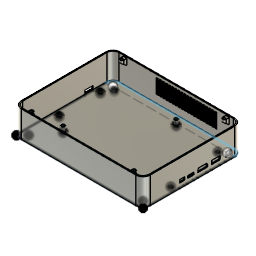
Mini PC Case V7 (Autodesk Fusion 360 design; units mm, degrees)
Autodesk Fusion 360 part; units mm, degrees
note: some values were not read from the file. Set by a fixed rule: which sketch regions a step uses.
sketch "Sketch1" plane through (0, 0, 0) normal (0, 0, 1) x (1, 0, 0)
  line L0 (10, 0) -> (200, 0)
  line L1 (210, 10) -> (210, 150)
  line L2 (210, 150) -> (0, 150) construction
  line L3 (0, 150) -> (0, 10)
  circle A0 centre (119, 146) radius 1.65
  circle A1 centre (191, 143) radius 1.65
  line L4 (-2, 152) -> (-2, 10)
  line L5 (10, -2) -> (200, -2)
  line L6 (212, 10) -> (212, 152)
  circle A2 centre (202, 54) radius 1.65
  circle A3 centre (34.7, 42.5) radius 1.65
  line L7 (210, 143.8) -> (212, 143.8)
  line L8 (210, 135.5) -> (212, 135.5)
  line L9 (210, 126) -> (212, 126)
  line L10 (210, 112) -> (212, 112)
  line L11 (210, 105) -> (212, 105)
  line L12 (210, 89) -> (212, 89)
  line L13 (210, 82.5) -> (212, 82.5)
  line L14 (210, 72) -> (212, 72)
  line L15 (210, 67) -> (212, 67)
  line L16 (210, 59) -> (212, 59)
  circle A4 centre (34.7, 42.5) radius 3
  circle A5 centre (202, 54) radius 3
  circle A6 centre (191, 143) radius 3
  circle A7 centre (119, 146) radius 3
  circle A8 centre (9, 130) radius 1.65
  circle A9 centre (8.6, 62) radius 1.65
  circle A10 centre (9, 130) radius 3
  circle A11 centre (8.6, 62) radius 3
  line L17 (0, 127) -> (-2, 127)
  line L18 (-2, 113.5) -> (0, 113.5)
  circle A12 centre (18, 144.2) radius 4
  line L19 (212, 152) -> (212, 150)
  line L20 (200, 162) -> (10, 162)
  line L21 (-2, 150) -> (-2, 152)
  line L22 (210, 152) -> (210, 150)
  line L23 (200, 160) -> (10, 160)
  line L24 (0, 150) -> (0, 152)
  line L25 (210, 150) -> (210, 152)
  line L26 (0, 150) -> (0, 152)
  arc A13 (200, 0) -> (210, 10) centre (200, 10) ccw
  arc A14 (210, 150) -> (200, 160) centre (200, 150) ccw
  arc A15 (10, 160) -> (0, 150) centre (10, 150) ccw
  arc A16 (0, 10) -> (10, 0) centre (10, 10) ccw
  arc A17 (-2, 10) -> (10, -2) centre (10, 10) ccw
  arc A18 (200, -2) -> (212, 10) centre (200, 10) ccw
  arc A19 (212, 150) -> (200, 162) centre (200, 150) ccw
  arc A20 (10, 162) -> (-2, 150) centre (10, 150) ccw
  point P0 (210, 0)
  dimension "d1" = 210
  dimension "d2" = 150
  dimension "d8" = 3.3
  dimension "d9" = 3.3
  dimension "d24" = 3.3
  dimension "d29" = 3.3
  dimension "d31" = 107.5
  dimension "d33" = 6.2
  dimension "d34" = 14.5
  dimension "d35" = 24
  dimension "d36" = 38
  dimension "d37" = 45
  dimension "d38" = 61
  dimension "d39" = 67.5
  dimension "d40" = 78
  dimension "d41" = 83
  dimension "d42" = 91
  dimension "d46" = 6
  dimension "d48" = 6
  dimension "d49" = 6
  dimension "d50" = 6
  dimension "d53" = 3.3
  dimension "d54" = 20
  dimension "d55" = 9
  dimension "d56" = 3.3
  dimension "d57" = 88
  dimension "d58" = 8.6
  dimension "d59" = 6
  dimension "d60" = 6
  dimension "d65" = 23
  dimension "d66" = 36.5
  dimension "d67" = 8
  dimension "d68" = 18
  dimension "d69" = 5.8
  dimension "d80" = 10
  dimension "d81" = 12
  dimension "d102" = 8
  dimension "d103" = 96
  dimension "d104" = 19
  dimension "d105" = 7
  dimension "d107" = 4
  dimension "d108" = 91
  dimension "d109" = 175.3
  constraint horizontal L0
  constraint vertical L1
  constraint horizontal L2
  constraint vertical L3
  constraint coincident L1 L7.start
  constraint coincident L6 L7.end
  constraint perpendicular L6 L7
  constraint coincident L1 L8.start
  constraint coincident L6 L8.end
  constraint perpendicular L6 L8
  constraint coincident L1 L9.start
  constraint coincident L6 L9.end
  constraint perpendicular L6 L9
  constraint coincident L1 L10.start
  constraint coincident L6 L10.end
  constraint perpendicular L6 L10
  constraint coincident L1 L11.start
  constraint coincident L6 L11.end
  constraint perpendicular L6 L11
  constraint coincident L1 L12.start
  constraint coincident L6 L12.end
  constraint perpendicular L6 L12
  constraint coincident L1 L13.start
  constraint coincident L6 L13.end
  constraint perpendicular L6 L13
  constraint coincident L1 L14.start
  constraint coincident L6 L14.end
  constraint perpendicular L6 L14
  constraint coincident L1 L15.start
  constraint coincident L6 L15.end
  constraint perpendicular L6 L15
  constraint coincident L1 L16.start
  constraint coincident L6 L16.end
  constraint perpendicular L6 L16
  constraint concentric A3 A4
  constraint concentric A2 A5
  constraint concentric A1 A6
  constraint concentric A0 A7
  constraint concentric A8 A10
  constraint concentric A9 A11
  constraint coincident L3 L17.start
  constraint coincident L4 L17.end
  constraint perpendicular L4 L17
  constraint coincident L4 L18.start
  constraint coincident L3 L18.end
  constraint perpendicular L3 L18
  constraint perpendicular L4 L20
  constraint perpendicular L3 L23
  constraint coincident P0 L0
  constraint coincident P0 L1
  constraint tangent L0 A13
  constraint tangent L1 A13
  constraint tangent L22 A14
  constraint tangent L23 A14
  constraint equal A13 A14
  constraint tangent L23 A15
  constraint tangent L24 A15
  constraint equal A13 A15
  constraint coincident origin L0
  constraint coincident origin L3
  constraint tangent L0 A16
  constraint tangent L3 A16
  constraint equal A13 A16
  constraint tangent L4 A17
  constraint tangent L5 A17
  constraint tangent L5 A18
  constraint tangent L6 A18
  constraint equal A17 A18
  constraint tangent L19 A19
  constraint tangent L20 A19
  constraint equal A17 A19
  constraint tangent L20 A20
  constraint tangent L21 A20
  constraint equal A17 A20
  measures "d1" distance of origin P0
  measures "d2" distance of origin L2.end
  measures "d8" diameter of A0
  measures "d9" diameter of A1
  measures "d24" diameter of A2
  measures "d29" diameter of A3
  measures "d31" distance of L2 A3.centre
  measures "d33" distance of L1.end L7
  measures "d34" distance of L1.end L8
  measures "d35" distance of L1.end L9
  measures "d36" distance of L1.end L10
  measures "d37" distance of L1.end L11
  measures "d38" distance of L1.end L12
  measures "d39" distance of L1.end L13
  measures "d40" distance of L1.end L14
  measures "d41" distance of L1.end L15
  measures "d42" distance of L1.end L16
  measures "d46" diameter of A4
  measures "d48" diameter of A5
  measures "d49" diameter of A6
  measures "d50" diameter of A7
  measures "d53" diameter of A8
  measures "d54" distance of L2 A8.centre
  measures "d55" distance of L3 A8.centre
  measures "d56" diameter of A9
  measures "d57" distance of L2 A9.centre
  measures "d58" distance of L3 A9.centre
  measures "d59" diameter of A10
  measures "d60" diameter of A11
  measures "d65" distance of L2 L17
  measures "d66" distance of L2 L18
  measures "d67" diameter of A12
  measures "d68" distance of L3 A12.centre
  measures "d69" distance of L2 A12.centre
  measures "d80" radius of A13
  measures "d81" radius of A17
  measures "d102" distance of L1 A2.centre
  measures "d103" distance of L2 A2.centre
  measures "d104" distance of L1 A1.centre
  measures "d105" distance of L2 A1.centre
  measures "d107" distance of L2 A0.centre
  measures "d108" distance of L1 A0.centre
  measures "d109" distance of L1 A3.centre
extrude "Extrude1" add sketch "Sketch1" along normal blind 2 contours L0 L1 L3 L23 A13 A14 A15 A16 | L0 L1 L3 L4 L5 L6 L16 L18 A13 A16 A17 A18 | L3 L4 L17 L18 | L1 L6 L15 L16 | L1 L3 L4 L6 L7 L17 L20 L23 A14 A15 A19 A20 | L1 L6 L14 L15 | L1 L6 L13 L14 | L1 L6 L12 L13 | L1 L6 L11 L12 | L1 L6 L10 L11 | L1 L6 L7 L8 | L1 L6 L9 L10 | L1 L6 L8 L9 | A0 | A1 | A2 | A3 | A4 | A5 | A6 | A7 | A8 | A9 | A10 | A11
extrude "Extrude2" add sketch "Sketch1" along normal blind 44 contours L0 L1 L3 L4 L5 L6 L16 L18 A13 A16 A17 A18 | L1 L3 L4 L6 L7 L17 L20 L23 A14 A15 A19 A20 | L1 L6 L14 L15 | L1 L6 L12 L13 | L1 L6 L10 L11 | L1 L6 L8 L9
extrude "Extrude3" add sketch "Sketch1" along normal blind 10 contours A4 | A5 | A6 | A7
extrude "Extrude4" add sketch "Sketch1" along normal blind 5 contours A10 | A11
extrude "Extrude8" add sketch "Sketch1" along normal blind 44 and the other way blind -8 contours L3 L4 L17 L18
extrude "Extrude9" add sketch "Sketch1" along normal blind 7 contours L1 L6 L7 L8
extrude "Extrude10" add sketch "Sketch1" along normal blind 8 contours L1 L6 L15 L16 | L1 L6 L13 L14 | L1 L6 L11 L12 | L1 L6 L9 L10
extrude "Extrude11" add sketch "Sketch1" along normal blind 14 and the other way blind -44 contours L1 L6 L11 L12 | L1 L6 L7 L8 | L1 L6 L9 L10
extrude "Extrude12" add 1 faces at (210.6667, 75.5, 8) along direction (0, 0, 1) blind 36 and the other way blind -4
extrude "Extrude13" add 1 faces at (210.6667, 64.3333, 8) along direction (0, 0, 1) blind 36 and the other way blind -5
fillet "Fillet1" radius 1 4 edges at (211, 82.5, 8) (211, 82.5, 12) (211, 72, 12) (211, 72, 8)
chamfer "Chamfer1" distance 1.5 angle 45 2 edges at (211, 105, 14) (211, 89, 14)
extrude "Extrude14" add 1 faces at (-0.6667, 118, 8) along direction (0, 0, -1) blind 6 and the other way blind -5
sketch "Sketch2" plane through (0, 160, 0) normal (0, -1, 0) x (1, 0, 0)
  line L0 (10, 2) -> (200, 2)
  line L1 (200, 2) -> (200, 44)
  line L2 (200, 44) -> (10, 44)
  line L3 (10, 44) -> (10, 2)
  line L4 (72, 39) -> (172, 39)
  line L5 (172, 39) -> (172, 15)
  line L6 (172, 15) -> (72, 15)
  line L7 (72, 15) -> (72, 39)
  line L8 (212, 13) -> (212, 8)
  line L9 (212, 8) -> (212, 13)
  line L10 (212, 8) -> (212, 9)
  line L11 (212, 8) -> (212, 9)
  line L12 (212, 9) -> (212, 11)
  line L13 (212, 11) -> (212, 12)
  line L14 (212, 11) -> (212, 12)
  line L15 (212, 11) -> (212, 9)
  line L16 (212, 12.5) -> (212, 8)
  line L17 (212, 8) -> (212, 12.5)
  line L18 (212, 12.5) -> (212, 14)
  line L19 (212, 14) -> (212, 12.5)
  line L20 (212, 14) -> (212, 8)
  line L21 (212, 8) -> (212, 14)
  line L22 (212, 44) -> (212, 0)
  line L23 (212, 0) -> (212, 44) construction
  line L24 (212, 14) -> (212, 7)
  line L25 (212, 7) -> (212, 14)
  line L26 (-2, 44) -> (-2, 0)
  line L27 (-2, 0) -> (-2, 44) construction
  line L28 (-2, 8) -> (-2, 3)
  line L29 (-2, 3) -> (-2, 8)
  line L30 (10, 0) -> (200, 0)
  line L31 (122, 39) -> (122, 15) construction
  line L32 (121, 39) -> (121, 15)
  line L33 (123, 39) -> (123, 15)
  line L34 (77, 39) -> (77, 15)
  line L35 (75, 39) -> (75, 15)
  line L36 (82.1111, 39) -> (82.1111, 15)
  line L37 (80.1111, 39) -> (80.1111, 15)
  line L38 (87.2222, 39) -> (87.2222, 15)
  line L39 (85.2222, 39) -> (85.2222, 15)
  line L40 (92.3333, 39) -> (92.3333, 15)
  line L41 (90.3333, 39) -> (90.3333, 15)
  line L42 (97.4444, 39) -> (97.4444, 15)
  line L43 (95.4444, 39) -> (95.4444, 15)
  line L44 (102.5556, 39) -> (102.5556, 15)
  line L45 (100.5556, 39) -> (100.5556, 15)
  line L46 (107.6667, 39) -> (107.6667, 15)
  line L47 (105.6667, 39) -> (105.6667, 15)
  line L48 (112.7778, 39) -> (112.7778, 15)
  line L49 (110.7778, 39) -> (110.7778, 15)
  line L50 (117.8889, 39) -> (117.8889, 15)
  line L51 (115.8889, 39) -> (115.8889, 15)
  line L52 (128.1111, 39) -> (128.1111, 15)
  line L53 (126.1111, 39) -> (126.1111, 15)
  line L54 (133.2222, 39) -> (133.2222, 15)
  line L55 (131.2222, 39) -> (131.2222, 15)
  line L56 (138.3333, 39) -> (138.3333, 15)
  line L57 (136.3333, 39) -> (136.3333, 15)
  line L58 (143.4444, 39) -> (143.4444, 15)
  line L59 (141.4444, 39) -> (141.4444, 15)
  line L60 (148.5556, 39) -> (148.5556, 15)
  line L61 (146.5556, 39) -> (146.5556, 15)
  line L62 (153.6667, 39) -> (153.6667, 15)
  line L63 (151.6667, 39) -> (151.6667, 15)
  line L64 (158.7778, 39) -> (158.7778, 15)
  line L65 (156.7778, 39) -> (156.7778, 15)
  line L66 (163.8889, 39) -> (163.8889, 15)
  line L67 (161.8889, 39) -> (161.8889, 15)
  line L68 (169, 39) -> (169, 15)
  line L69 (167, 39) -> (167, 15)
  dimension "d117" = 40
  dimension "d118" = 140
  dimension "d119" = 5
  dimension "d120" = 15
  dimension "d121" = 1
  dimension "d122" = 1
  dimension "d125" = 46
  dimension "d126" = 0
  constraint horizontal L4
  constraint vertical L5
  constraint horizontal L6
  constraint vertical L7
  constraint midpoint L4 L31.start
  constraint midpoint L6 L31.end
  constraint coincident L4 L32.start
  constraint coincident L6 L32.end
  constraint perpendicular L6 L32
  constraint coincident L4 L33.start
  constraint coincident L6 L33.end
  constraint perpendicular L6 L33
  measures "d117" distance of L5 L23
  measures "d118" distance of L7 L23
  measures "d119" distance of L2 L4
  measures "d120" distance of L6 L30
  measures "d121" distance of L31 L32
  measures "d122" distance of L31 L33
extrude "Extrude15" cut sketch "Sketch2" against normal up to surface (2 mm away) contours L4 L6 L7 L35 | L4 L6 L34 L37 | L4 L6 L36 L39 | L4 L6 L38 L41 | L4 L6 L40 L43 | L4 L6 L42 L45 | L4 L6 L44 L47 | L4 L6 L46 L49 | L4 L6 L48 L51 | L4 L6 L32 L50 | L4 L6 L33 L53 | L4 L6 L52 L55 | L4 L6 L54 L57 | L4 L6 L56 L59 | L4 L6 L58 L61 | L4 L6 L60 L63 | L4 L6 L62 L65 | L4 L6 L64 L67 | L4 L6 L66 L69 | L4 L5 L6 L68
sketch "Sketch3" plane through (0, 0, 44) normal (0, 0, 1) x (-1, 0, 0)
  line L0 (-212, -10) -> (-212, -150)
  arc A0 (-212, -150) -> (-200, -162) centre (-200, -150) ccw
  line L1 (-200, -162) -> (-10, -162)
  arc A1 (-10, -162) -> (2, -150) centre (-10, -150) ccw
  line L2 (2, -150) -> (2, -10)
  arc A2 (2, -10) -> (-10, 2) centre (-10, -10) ccw
  line L3 (-10, 2) -> (-200, 2)
  arc A3 (-200, 2) -> (-212, -10) centre (-200, -10) ccw
  line L4 (-210, -150) -> (-210, -10)
  arc A4 (-200, 0) -> (-210, -10) centre (-200, -10) ccw
  line L5 (-200, 0) -> (-10, 0)
  arc A5 (0, -10) -> (-10, 0) centre (-10, -10) ccw
  line L6 (0, -10) -> (0, -150)
  arc A6 (-10, -160) -> (0, -150) centre (-10, -150) ccw
  line L7 (-10, -160) -> (-200, -160)
  arc A7 (-210, -150) -> (-200, -160) centre (-200, -150) ccw
  circle A8 centre (-20, -5) radius 1.65
  circle A9 centre (-20, -5) radius 3
  line L8 (-10, 0) -> (-200, 0)
  line L9 (0, -150) -> (0, -10)
  line L10 (0, -80) -> (-210, -80) construction
  line L11 (-105, -160) -> (-105, 0) construction
  line L12 (-17, -5) -> (-17, 0)
  line L13 (-23, -5) -> (-23, 0)
  dimension "d129" = 3.3
  dimension "d130" = 6
  dimension "d131" = 5
  dimension "d132" = 5
  dimension "d133" = 20
  dimension "d134" = 20
  constraint midpoint L9 L10.start
  constraint midpoint L4 L10.end
  constraint midpoint L7 L11.start
  constraint midpoint L8 L11.end
  constraint coincident A9 L12.start
  constraint coincident L8 L12.end
  constraint perpendicular L8 L12
  constraint coincident A9 L13.start
  constraint coincident L8 L13.end
  constraint perpendicular L8 L13
  measures "d129" diameter of A8
  measures "d130" diameter of A9
  measures "d131" distance of A8.centre L8
  measures "d132" distance of A8.centre L8
  measures "d133" distance of A8.centre L9
  measures "d134" distance of A8.centre L9
extrude "Extrude16" add sketch "Sketch3" along normal blind -12 and the other way blind 2 contours L5 A9 L8 L12 L13 | A9 | A8
sketch "Sketch4" plane through (23, 0, 0) normal (1, 0, 0) x (0, 1, 0)
  line L0 (5, 42) -> (0, 42)
  line L1 (0, 42) -> (0, 32)
  line L2 (0, 32) -> (5, 32)
  line L3 (5, 32) -> (5, 42)
  line L4 (5, 42) -> (8, 42)
  line L5 (5, 42) -> (5, 32)
  line L6 (5, 32) -> (8, 32)
  line L7 (5, 32) -> (5, 42)
  line L8 (0, 32) -> (8, 38)
  line L9 (8, 38) -> (8, 32)
  line L10 (0, 32) -> (8, 32)
  line L11 (8, 42) -> (8, 32) construction
  dimension "d143" = 6
  constraint coincident L1.end L2.start
  constraint coincident L6.end L9.end
  constraint coincident L4.end L11.start
  constraint coincident L8.end L11
  measures "d143" distance of L8.end L6.end
extrude "Extrude17" cut sketch "Sketch4" against normal blind 7 contours L3 L5 L6 L7 L8 L9 L10 | L2 L3 L5 L7 L8 L10
extrude "Extrude18" cut sketch "Sketch3" against normal blind 6 contours A8
ref_plane "WorkPlane1" through (105, 80, 23) normal (1, 0, 0) x (0, 1, 0)
ref_plane "WorkPlane2" through (105, 80, 23) normal (0, -1, 0) x (1, 0, 0)
mirror "Mirror1" about plane through (105, 80, 23) normal (1, 0, 0) of "Extrude16", "Extrude17", "Extrude18"
mirror "Mirror2" about plane through (105, 80, 23) normal (0, -1, 0) of "Extrude16", "Extrude17", "Extrude18", "Mirror1"
equation "d8 = HolesRadius"
equation "d9 = HolesRadius"
equation "d24 = HolesRadius"
equation "d29 = HolesRadius"
equation "HolesRadius = 3.3 mm"
equation "d46 = HolesOuterRadius"
equation "HolesOuterRadius = 6 mm"
equation "d48 = HolesOuterRadius"
equation "d49 = HolesOuterRadius"
equation "d50 = HolesOuterRadius"
equation "d53 = HolesRadius"
equation "d56 = HolesRadius"
equation "d59 = HolesOuterRadius"
equation "d60 = HolesOuterRadius"
equation "d129 = HolesRadius"
equation "d130 = HolesOuterRadius"
